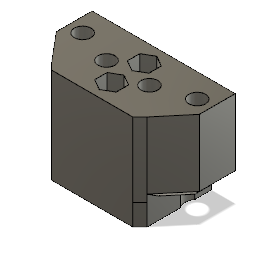
Hanger__Ceiling__Interchange (Autodesk Fusion 360 design; units mm, degrees)
Autodesk Fusion 360 part; units mm, degrees
sketch "Sketch1" plane through (0, 0, 0) normal (0, 1, 0) x (1, 0, 0)
  line L0 (0, 0) -> (60, 0)
  line L1 (60, 0) -> (60, -40)
  line L2 (60, -40) -> (0, -40)
  line L3 (0, -40) -> (0, 0)
  dimension "d1" = 60
  dimension "d2" = 40
  constraint horizontal L0
  constraint vertical L1
  constraint horizontal L2
  constraint vertical L3
  constraint coincident L0.start L3.end
  measures "d1" distance of L0.start L0.end
  measures "d2" distance of L0.start L2.end
extrude "Extrude1" add sketch "Sketch1" along normal blind 25
sketch "Sketch2" plane through (0, 25, 0) normal (0, 1, 0) x (-1, 0, 0)
  line L0 (0, 40) -> (-60, 40)
  line L1 (-60, 40) -> (-60, 0)
  line L2 (-60, 0) -> (0, 0)
  line L3 (0, 0) -> (0, 40)
  line L4 (-30, 0) -> (-30, 20)
  line L5 (-30, 20) -> (-39, 20)
  line L6 (-30, 20) -> (-21, 20)
  line L7 (-21, 20) -> (-6, 20)
  line L8 (-39, 20) -> (-54, 20)
  circle A0 centre (-21, 20) radius 3.5
  circle A1 centre (-39, 20) radius 3.5
  circle A2 centre (-54, 20) radius 3.5
  circle A3 centre (-6, 20) radius 3.5
  dimension "d5" = 20
  dimension "d6" = 9
  dimension "d7" = 9
  dimension "d8" = 15
  dimension "d9" = 15
  dimension "d10" = 7
  dimension "d11" = 7
  dimension "d12" = 7
  dimension "d13" = 7
  constraint midpoint L2 L4.start
  constraint perpendicular L0 L4
  constraint perpendicular L4 L5
  constraint perpendicular L4 L6
  constraint parallel L6 L7
  constraint perpendicular L4 L8
  constraint coincident L6.end L7.start
  constraint coincident L5.end L8.start
  constraint coincident L8.end A2.centre
  constraint coincident L7.end A3.centre
  measures "d5" distance of L4.start L4.end
  measures "d6" distance of L4.end L5.end
  measures "d7" distance of L4.end L6.end
  measures "d8" distance of L6.end L7.end
  measures "d9" distance of L5.end L8.end
  measures "d10" diameter of A0
  measures "d11" diameter of A1
  measures "d12" diameter of A2
  measures "d13" diameter of A3
extrude "Extrude2" cut sketch "Sketch2" against normal blind 25 contours L5 L8 A1 | L5 L8 A1 | L6 L7 A0 | L6 L7 A0 | A2 | A3
sketch "Sketch3" plane through (0, 0, 0) normal (0, -1, 0) x (1, 0, 0)
  circle A0 centre (21, 20) radius 3.5
  circle A1 centre (39, 20) radius 3.5
  circle A2 centre (6, 20) radius 3.5
  circle A3 centre (54, 20) radius 3.5
  line L0 (60, 40) -> (0, 40)
  line L1 (0, 40) -> (0, 0)
  line L2 (0, 0) -> (60, 0)
  line L3 (60, 0) -> (60, 40)
  circle A4 centre (6, 20) radius 6.5
  circle A5 centre (21, 20) radius 6.5
  circle A6 centre (39, 20) radius 6.5
  circle A7 centre (54, 20) radius 6.5
  dimension "d16" = 13
  dimension "d17" = 13
  dimension "d18" = 13
  dimension "d19" = 13
  constraint concentric A2 A4
  constraint concentric A0 A5
  constraint concentric A1 A6
  constraint concentric A3 A7
  measures "d16" diameter of A4
  measures "d17" diameter of A5
  measures "d18" diameter of A6
  measures "d19" diameter of A7
extrude "Extrude3" cut sketch "Sketch3" against normal blind 2 contours L3 A7 | L1 A4 | A5 | A6 picked at (59.1667, 20) picked at (0.8333, 20)
extrude "Extrude4" cut 4 faces at (0.8333, 2, 20) (26.4628, 2, 19.5032) (44.4758, 2, 19.6771) (59.1667, 2, 20) along direction (0, 1, 0) blind 13
sketch "Sketch4" plane through (0, 25, 0) normal (0, 1, 0) x (-1, 0, 0)
  circle A0 centre (-21, 20) radius 3.5
  circle A1 centre (-39, 20) radius 3.5
  circle A2 centre (-6, 20) radius 3.5
  circle A3 centre (-54, 20) radius 3.5
  line L0 (0, 40) -> (-60, 40)
  line L1 (-60, 40) -> (-60, 0)
  line L2 (-60, 0) -> (0, 0)
  line L3 (0, 0) -> (0, 40)
  line L4 (-30, 40) -> (-30, 0)
  line L5 (-30, 20) -> (-30, 26.85)
  line L6 (-30, 26.85) -> (-30, 13.15)
  circle A4 centre (-30, 13.15) radius 2
  circle A5 centre (-30, 26.85) radius 2
  dimension "d24" = 6.85
  dimension "d25" = 13.7
  dimension "d26" = 4
  dimension "d27" = 4
  constraint midpoint L0 L4.start
  constraint midpoint L2 L4.end
  constraint midpoint L4 L5.start
  constraint parallel L4 L5
  constraint parallel L4 L6
  constraint coincident L6.end A4.centre
  constraint coincident L5.end L6.start
  measures "d24" distance of L5.start L5.end
  measures "d25" distance of L5.end L6.end
  measures "d26" diameter of A4
  measures "d27" diameter of A5
sketch "Sketch5" plane through (0, 25, 0) normal (0, 1, 0) x (-1, 0, 0)
  circle A0 centre (-21, 20) radius 3.5
  circle A1 centre (-39, 20) radius 3.5
  circle A2 centre (-6, 20) radius 3.5
  circle A3 centre (-54, 20) radius 3.5
  line L0 (0, 40) -> (-60, 40)
  line L1 (-60, 40) -> (-60, 0)
  line L2 (-60, 0) -> (0, 0)
  line L3 (0, 0) -> (0, 40)
  line L4 (-34.5, 24.2519) -> (-30, 21.6538)
  line L5 (-30, 21.6538) -> (-25.5, 24.2519)
  line L6 (-25.5, 24.2519) -> (-25.5, 29.4481)
  line L7 (-25.5, 29.4481) -> (-30, 32.0462)
  line L8 (-30, 32.0462) -> (-34.5, 29.4481)
  line L9 (-34.5, 29.4481) -> (-34.5, 24.2519)
  line L10 (-34.5, 10.5519) -> (-30, 7.9538)
  line L11 (-30, 7.9538) -> (-25.5, 10.5519)
  line L12 (-25.5, 10.5519) -> (-25.5, 15.7481)
  line L13 (-25.5, 15.7481) -> (-30, 18.3462)
  line L14 (-30, 18.3462) -> (-34.5, 15.7481)
  line L15 (-34.5, 15.7481) -> (-34.5, 10.5519)
  point P0 (-30, 26.85)
  point P1 (-30, 13.15)
  dimension "d30" = 4.5
  dimension "d31" = 4.5
  measures "d30" distance of P0 L9
  measures "d31" distance of P1 L15
sketch "Sketch6" plane through (0, 0, 0) normal (0, -1, 0) x (1, 0, 0)
  arc A0 (60, 22.5) -> (60, 17.5) centre (54, 20) ccw
  line L0 (60, 22.5) -> (60, 40)
  line L1 (60, 40) -> (0, 40)
  line L2 (0, 40) -> (0, 22.5)
  arc A1 (0, 17.5) -> (0, 22.5) centre (6, 20) ccw
  line L3 (0, 17.5) -> (0, 0)
  line L4 (0, 0) -> (60, 0)
  line L5 (60, 0) -> (60, 17.5)
  circle A2 centre (21, 20) radius 6.5
  circle A3 centre (39, 20) radius 6.5
  circle A4 centre (6, 20) radius 5
  circle A5 centre (21, 20) radius 5
  circle A6 centre (54, 20) radius 5
  circle A7 centre (39, 20) radius 5
  circle A8 centre (6, 20) radius 6.5
  circle A9 centre (54, 20) radius 6.5
  circle A10 centre (39, 20) radius 6.5
  circle A11 centre (21, 20) radius 6.5
  dimension "d32" = 10
  dimension "d33" = 10
  dimension "d34" = 10
  dimension "d35" = 10
  constraint concentric A1 A4
  constraint concentric A2 A5
  constraint concentric A0 A6
  constraint concentric A3 A7
  constraint concentric A4 A8
  constraint concentric A6 A9
  constraint concentric A7 A10
  constraint concentric A5 A11
  measures "d32" diameter of A4
  measures "d33" diameter of A5
  measures "d34" diameter of A6
  measures "d35" diameter of A7
extrude "Extrude6" add sketch "Sketch6" against normal blind 15 contours A0 A9 | A1 A8 | A2 A11 | A3 A10
sketch "Sketch7" plane through (0, 25, 0) normal (0, 1, 0) x (-1, 0, 0)
  circle A0 centre (-21, 20) radius 3.5
  circle A1 centre (-39, 20) radius 3.5
  circle A2 centre (-6, 20) radius 3.5
  circle A3 centre (-54, 20) radius 3.5
  line L0 (0, 40) -> (-60, 40)
  line L1 (-60, 40) -> (-60, 0)
  line L2 (-60, 0) -> (0, 0)
  line L3 (0, 0) -> (0, 40)
  line L4 (-60, 40) -> (0, 40)
  line L5 (0, 40) -> (0, 0)
  line L6 (0, 0) -> (-60, 0)
  line L7 (-60, 0) -> (-60, 40)
  line L8 (-63.5098, 43.7878) -> (2.9374, 43.7878)
  line L9 (2.9374, 43.7878) -> (2.9374, -3.4155)
  line L10 (2.9374, -3.4155) -> (-63.5098, -3.4155)
  line L11 (-63.5098, -3.4155) -> (-63.5098, 43.7878)
  constraint horizontal L4
  constraint vertical L5
  constraint horizontal L6
  constraint vertical L7
  constraint coincident L2.end L3.start
  constraint coincident L0.end L1.start
  constraint horizontal L8
  constraint vertical L9
  constraint horizontal L10
  constraint vertical L11
extrude "Extrude8" cut sketch "Sketch7" against normal blind 41 contours L8 L9 L10 L11
sketch "Sketch8" plane through (0, 0, 0) normal (-1, 0, 0) x (0, 0, 1)
  line L0 (0, 0) -> (40, 0)
  line L1 (40, 0) -> (40, 25)
  line L2 (40, 25) -> (0, 25)
  line L3 (0, 25) -> (0, 0)
  line L4 (40, 0) -> (37, 0)
  line L5 (40, 0) -> (40, 3)
  line L6 (40, 3) -> (37, 0)
  dimension "d42" = 3
  dimension "d43" = 3
  constraint coincident L0.end L1.start
  constraint perpendicular L1 L4
  constraint perpendicular L0 L5
  measures "d42" distance of L0.end L4.end
  measures "d43" distance of L0.end L5.end
extrude "Extrude9" cut sketch "Sketch8" against normal blind 10 contours L0 L1 L4 L5 L6
extrude "Extrude10" cut 1 faces at (10, 1, 39) along direction (-1, 0, 0) blind -40 and the other way blind 50
sketch "Sketch9" plane through (0, 25, 0) normal (0, 1, 0) x (-1, 0, 0)
  circle A0 centre (-21, 20) radius 3.5
  circle A1 centre (-39, 20) radius 3.5
  circle A2 centre (-6, 20) radius 3.5
  circle A3 centre (-54, 20) radius 3.5
  line L0 (0, 40) -> (-60, 40)
  line L1 (-60, 40) -> (-60, 0)
  line L2 (-60, 0) -> (0, 0)
  line L3 (0, 0) -> (0, 40)
  line L4 (-30, 40) -> (-30, 31.85)
  circle A4 centre (-30, 31.85) radius 2
  line L5 (-30, 31.85) -> (-30, 18.15)
  circle A5 centre (-30, 18.15) radius 2
  dimension "d50" = 8.15
  dimension "d51" = 4
  dimension "d52" = 13.7
  dimension "d53" = 4
  constraint midpoint L0 L4.start
  constraint perpendicular L0 L4
  constraint coincident L4.end A4.centre
  constraint parallel L4 L5
  constraint coincident L5.end A5.centre
  measures "d50" distance of L4.start L4.end
  measures "d51" diameter of A4
  measures "d52" distance of L4.end L5.end
  measures "d53" diameter of A5
extrude "Extrude11" cut sketch "Sketch9" against normal blind 25 contours L4 A4 L5 | L4 A4 L5 | A5
sketch "Sketch10" plane through (0, 25, 0) normal (0, 1, 0) x (-1, 0, 0)
  circle A0 centre (-30, 31.85) radius 2
  circle A1 centre (-30, 18.15) radius 2
  circle A2 centre (-21, 20) radius 3.5
  circle A3 centre (-39, 20) radius 3.5
  circle A4 centre (-6, 20) radius 3.5
  circle A5 centre (-54, 20) radius 3.5
  line L0 (0, 40) -> (-60, 40)
  line L1 (-60, 40) -> (-60, 0)
  line L2 (-60, 0) -> (0, 0)
  line L3 (0, 0) -> (0, 40)
  line L4 (-34.5, 29.2519) -> (-30, 26.6538)
  line L5 (-30, 26.6538) -> (-25.5, 29.2519)
  line L6 (-25.5, 29.2519) -> (-25.5, 34.4481)
  line L7 (-25.5, 34.4481) -> (-30, 37.0462)
  line L8 (-30, 37.0462) -> (-34.5, 34.4481)
  line L9 (-34.5, 34.4481) -> (-34.5, 29.2519)
  line L10 (-34.5, 15.5519) -> (-30, 12.9538)
  line L11 (-30, 12.9538) -> (-25.5, 15.5519)
  line L12 (-25.5, 15.5519) -> (-25.5, 20.7481)
  line L13 (-25.5, 20.7481) -> (-30, 23.3462)
  line L14 (-30, 23.3462) -> (-34.5, 20.7481)
  line L15 (-34.5, 20.7481) -> (-34.5, 15.5519)
  point P0 (-30, 31.85)
  point P1 (-30, 18.15)
  dimension "d56" = 4.5
  dimension "d57" = 4.5
  constraint coincident P0 A0.centre
  constraint coincident P1 A1.centre
  measures "d56" distance of P0 L9
  measures "d57" distance of P1 L15
extrude "Extrude12" cut sketch "Sketch10" against normal blind 15 contours L4 L5 L6 L7 L8 L9 | L10 L11 L12 L13 L14 L15
sketch "Sketch11" plane through (0, 0, 0) normal (0, -1, 0) x (1, 0, 0)
sketch "Sketch12" plane through (0, 0, 40) normal (0, 0, 1) x (1, 0, 0)
sketch "Sketch13" plane through (0, 0, 0) normal (0, -1, 0) x (1, 0, 0)
sketch "Sketch14" plane through (0, 0, 40) normal (0, 0, 1) x (1, 0, 0)
ref_plane "WorkPlane1" through (11.5, 0, 38.5) normal (-0.579228, -0.573576, 0.579228) x (-0.707107, 0, -0.707107)
sketch "Sketch15" plane through (11.5, 0, 38.5) normal (-0.579228, -0.573576, 0.579228) x (-0.707107, 0, -0.707107)
  line L0 (2.1213, 0, 0) -> (0, -3.6742, 0.017)
  line L1 (0, -3.6742, 0.017) -> (-2.1213, 0, 0)
  line L2 (-2.1213, 0) -> (2.1213, 0)
  point P0 (2.1213, 0)
  point P1 (0, -3.6742)
  point P2 (-2.1213, 0)
  constraint coincident P0 L2.end
  constraint coincident P2 L2.start
extrude "Extrude13" cut sketch "Sketch15" along normal blind 5 contours L0 L1 L2 in plane through (11.5, 0, 38.5) normal (-0.57735, -0.57735, 0.57735)
ref_plane "WorkPlane2" through (48.5, 1.5, 40) normal (0.579228, -0.579228, 0.573576) x (0.707107, 0.707107, 0)
sketch "Sketch16" plane through (48.5, 1.5, 40) normal (0.579228, -0.579228, 0.573576) x (0.707107, 0.707107, 0)
  line L0 (-2.1213, 0) -> (2.1213, 0)
  line L1 (2.1213, 0, 0) -> (0, -3.6742, 0.017)
  line L2 (0, -3.6742, 0.017) -> (-2.1213, 0, 0)
  point P0 (-2.1213, 0)
  point P1 (2.1213, 0)
  point P2 (0, -3.6742)
  constraint coincident P0 L0.start
  constraint coincident P1 L0.end
extrude "Extrude14" cut sketch "Sketch16" along normal blind 5 contours L0 L1 L2 in plane through (48.5, 1.5, 40) normal (0.57735, -0.57735, 0.57735)
chamfer "Chamfer1" distance 3 distance2 3 2 edges at (0, 14, 40) (60, 14, 40) measured on face at (0, 16.6667, 25.6667) measured on face at (23.3333, 17.6667, 40)
chamfer "Chamfer2" distance 3 angle 45 1 edges at (60, 0, 18.5)
chamfer "Chamfer3" distance 3 angle 45 1 edges at (0, 0, 18.5)
extrude "Extrude15" add 1 faces at (30, 25, 4.3179) along direction (0, 1, 0) blind 15
extrude "Extrude16" add 2 faces at (28.1667, 10, 28.6746) (28.1667, 10, 14.9746) along direction (0, 1, 0) blind 15
extrude "Extrude17" cut 4 faces at (10.4684, 15, 19.5777) (25.1536, 15, 19.349) (34.8464, 15, 19.349) (58.4684, 15, 19.5777) along direction (0, 1, 0) blind 15
extrude "Extrude18" cut 1 faces at (39, 26.6667, 0) along direction (0, 0, 1) blind 5
sketch "Sketch17" plane through (0, 0, 0) normal (0, -1, 0) x (1, 0, 0)
  line L0 (3, 5) -> (57, 5)
  line L1 (57, 5) -> (57, 16)
  arc A0 (57, 24) -> (57, 16) centre (54, 20) ccw
  line L2 (57, 24) -> (57, 37)
  line L3 (57, 37) -> (50, 37)
  line L4 (50, 37) -> (47, 40)
  line L5 (47, 40) -> (13, 40)
  line L6 (13, 40) -> (10, 37)
  line L7 (10, 37) -> (3, 37)
  line L8 (3, 37) -> (3, 24)
  arc A1 (3, 16) -> (3, 24) centre (6, 20) ccw
  line L9 (3, 16) -> (3, 5)
  circle A2 centre (30, 31.85) radius 2
  circle A3 centre (30, 18.15) radius 2
  circle A4 centre (21, 20) radius 5
  circle A5 centre (39, 20) radius 5
  line L10 (50, 37) -> (50, 54.6936)
  line L11 (50, 37) -> (50, 40)
  line L12 (50, 40) -> (62.2647, 25.3835)
  line L13 (62.2647, 25.3835) -> (62.2647, 41)
  line L14 (62.2647, 41) -> (50, 41)
  line L15 (10, 37) -> (10, 40)
  line L16 (10, 40) -> (-2.3313, 25.3041)
  line L17 (-2.3313, 25.3041) -> (-2.3313, 43)
  line L18 (-2.3313, 43) -> (10, 43)
  line L19 (10, 43) -> (10, 40)
  dimension "d81" = 40
  dimension "d82" = 40
  constraint coincident L3.end L4.start
  constraint perpendicular L3 L10
  constraint coincident L10 L11.end
  constraint parallel L11 L13
  constraint coincident L10 L14.end
  constraint perpendicular L10 L14
  constraint coincident L6.end L7.start
  constraint perpendicular L7 L15
  constraint perpendicular L7 L17
  constraint perpendicular L15 L18
  constraint perpendicular L18 L19
  measures "d81" angle of L11 L12
  measures "d82" angle of L15 L16
extrude "Extrude19" cut sketch "Sketch17" against normal blind 50 contours L7 L8 L16 L17 L18 L19 | L7 L8 L16 | L2 L3 L12 | L2 L3 L10 L12 L13 L14
sketch "Sketch18" plane through (60, 0, 0) normal (1, 0, 0) x (0, 0, -1)
  line L0 (-28.0825, 40) -> (-28.0825, 3)
  line L1 (-28.0825, 3) -> (-5, 3)
  line L2 (-5, 3) -> (-5, 40)
  line L3 (-5, 40) -> (-28.0825, 40)
  line L4 (-5, 0) -> (-40, 0)
  line L5 (-40, 0) -> (-40, 9)
  line L6 (-40, 9) -> (-5, 9)
  line L7 (-5, 9) -> (-5, 0)
  dimension "d85" = 9
  constraint horizontal L4
  constraint vertical L5
  constraint horizontal L6
  constraint vertical L7
  measures "d85" distance of L4.start L6.end
extrude "Extrude20" cut sketch "Sketch18" against normal blind 5 contours L0 L1 L2 L6 L7 | L0 L1 L4 L5 L6 L7
sketch "Sketch19" plane through (0, 0, 0) normal (-1, 0, 0) x (0, 0, 1)
  line L0 (28.0825, 3) -> (28.0825, 40)
  line L1 (28.0825, 40) -> (5, 40)
  line L2 (5, 40) -> (5, 3)
  line L3 (5, 3) -> (28.0825, 3)
  line L4 (5, 0) -> (40, 0)
  line L5 (40, 0) -> (40, 9)
  line L6 (40, 9) -> (5, 9)
  line L7 (5, 9) -> (5, 0)
  dimension "d88" = 35
  dimension "d89" = 9
  constraint horizontal L4
  constraint vertical L5
  constraint horizontal L6
  constraint vertical L7
  measures "d88" distance of L4.start L4.end
  measures "d89" distance of L4.start L6.end
extrude "Extrude21" cut sketch "Sketch19" against normal blind 5 contours L0 L2 L3 L6 L7 | L0 L3 L4 L5 L6 L7
sketch "Sketch20" plane through (0, 0, 0) normal (0, -1, 0) x (1, 0, 0)
  line L0 (5, 15.101) -> (5, 5)
  line L1 (5, 5) -> (55, 5)
  line L2 (55, 5) -> (55, 15.101)
  arc A0 (55, 24.899) -> (55, 15.101) centre (54, 20) ccw
  line L3 (55, 24.899) -> (55, 34.0412)
  line L4 (55, 34.0412) -> (52.5173, 37)
  line L5 (52.5173, 37) -> (50, 37)
  line L6 (50, 37) -> (47, 40)
  line L7 (47, 40) -> (13, 40)
  line L8 (13, 40) -> (10, 37)
  line L9 (10, 37) -> (7.4827, 37)
  line L10 (7.4827, 37) -> (5, 34.0412)
  line L11 (5, 34.0412) -> (5, 24.899)
  arc A1 (5, 15.101) -> (5, 24.899) centre (6, 20) ccw
  circle A2 centre (30, 31.85) radius 2
  circle A3 centre (30, 18.15) radius 2
  circle A4 centre (21, 20) radius 5
  circle A5 centre (39, 20) radius 5
  line L12 (50, 37) -> (50, 5)
  line L13 (10, 37) -> (10, 5)
  line L14 (10, 5) -> (2, 5)
  line L15 (2, 5) -> (2, 40)
  line L16 (2, 40) -> (10, 40)
  line L17 (10, 40) -> (10, 5)
  line L18 (50, 5) -> (57, 5)
  line L19 (57, 5) -> (57, 40)
  line L20 (57, 40) -> (50, 40)
  line L21 (50, 40) -> (50, 5)
  constraint coincident L5.end L6.start
  constraint coincident L1 L12.end
  constraint perpendicular L1 L12
  constraint coincident L8.end L9.start
  constraint coincident L1 L13.end
  constraint perpendicular L1 L13
  constraint horizontal L14
  constraint vertical L15
  constraint horizontal L16
  constraint vertical L17
  constraint horizontal L18
  constraint vertical L19
  constraint horizontal L20
  constraint vertical L21
extrude "Extrude22" cut sketch "Sketch20" against normal blind 9 contours L0 L1 A1 L13 L14 L17 | L0 L9 L10 L11 A1 L13 L14 L15 L16 L17 | L9 L10 L11 A1 L13 L17 | L1 L2 A0 L12 L18 L21 | L2 A0 L3 L4 L5 L12 L18 L19 L20 L21 | A0 L3 L4 L5 L12 L21
sketch "Sketch21" plane through (0, 0, 40) normal (0, 0, 1) x (1, 0, 0)
  line L0 (10, 40) -> (10, 9)
  line L1 (10, 9) -> (10, 3)
  line L2 (10, 3) -> (13, 0)
  line L3 (13, 0) -> (47, 0)
  line L4 (47, 0) -> (50, 3)
  line L5 (50, 3) -> (50, 9)
  line L6 (50, 9) -> (50, 40)
  line L7 (50, 40) -> (10, 40)
  line L8 (10, 0) -> (14, 0)
  line L9 (14, 0) -> (14, 3)
  line L10 (14, 3) -> (10, 3)
  line L11 (10, 3) -> (10, 0)
  line L12 (50, 0) -> (47, 0)
  line L13 (47, 0) -> (47, 3.1875)
  line L14 (47, 3.1875) -> (50, 3.1875)
  line L15 (50, 3.1875) -> (50, 0)
  constraint horizontal L8
  constraint vertical L9
  constraint horizontal L10
  constraint vertical L11
  constraint horizontal L12
  constraint vertical L13
  constraint horizontal L14
  constraint vertical L15
extrude "Extrude23" add sketch "Sketch21" against normal blind 3 contours L2 L8 L11 | L4 L12 L15
chamfer "Chamfer5" distance 3 angle 45 2 edges at (10, 4.5, 40) (50, 4.5, 40)
sketch "Sketch22" plane through (0, 0, 0) normal (0, -1, 0) x (1, 0, 0)
  circle A0 centre (39, 20) radius 5
  circle A1 centre (21, 20) radius 5
  circle A2 centre (30, 18.15) radius 2
  circle A3 centre (30, 31.85) radius 2
  line L0 (50, 37) -> (47, 40)
  line L1 (47, 40) -> (13, 40)
  line L2 (13, 40) -> (10, 37)
  line L3 (10, 37) -> (10, 23)
  arc A4 (10, 17) -> (10, 23) centre (6, 20) ccw
  line L4 (10, 17) -> (10, 5)
  line L5 (10, 5) -> (50, 5)
  line L6 (50, 5) -> (50, 17)
  arc A5 (50, 23) -> (50, 17) centre (54, 20) ccw
  line L7 (50, 23) -> (50, 37)
  line L8 (10, 37) -> (0, 28)
  line L9 (50, 37) -> (60, 28)
  line L10 (0, 28) -> (60, 28)
  line L11 (60, 28) -> (60, 40)
  line L12 (60, 40) -> (0, 40)
  line L13 (0, 40) -> (0, 28)
  line L14 (10, 37) -> (13, 37)
  line L15 (13, 37) -> (13, 40)
  line L16 (13, 40) -> (10, 40)
  line L17 (10, 40) -> (10, 37)
  line L18 (50, 37) -> (47, 37)
  line L19 (47, 37) -> (47, 40)
  line L20 (47, 40) -> (50, 40)
  line L21 (50, 40) -> (50, 37)
  constraint coincident L2.end L3.start
  constraint coincident L0.start L7.end
  constraint horizontal L10
  constraint vertical L11
  constraint horizontal L12
  constraint vertical L13
  constraint horizontal L14
  constraint vertical L15
  constraint horizontal L16
  constraint vertical L17
  constraint coincident L1.end L2.start
  constraint horizontal L18
  constraint vertical L19
  constraint horizontal L20
  constraint vertical L21
  constraint coincident L0.end L1.start
extrude "Extrude24" cut sketch "Sketch22" against normal blind 100 contours L9 L11 L12 L21 | L0 L12 L20 L21 | L2 L12 L16 L17 | L8 L12 L13 L17
sketch "Sketch23" plane through (0, 0, 0) normal (0, -1, 0) x (1, 0, 0)
  circle A0 centre (39, 20) radius 5
  circle A1 centre (21, 20) radius 5
  circle A2 centre (30, 18.15) radius 2
  circle A3 centre (30, 31.85) radius 2
  line L0 (50, 37) -> (47, 40)
  line L1 (47, 40) -> (13, 40)
  line L2 (13, 40) -> (10, 37)
  line L3 (10, 37) -> (10, 23)
  arc A4 (10, 17) -> (10, 23) centre (6, 20) ccw
  line L4 (10, 17) -> (10, 5)
  line L5 (10, 5) -> (50, 5)
  line L6 (50, 5) -> (50, 17)
  arc A5 (50, 23) -> (50, 17) centre (54, 20) ccw
  line L7 (50, 23) -> (50, 37)
  line L8 (50, 37) -> (62.7874, 21.7606)
  line L9 (50, 37) -> (69.8936, 37) construction
  line L10 (10, 37) -> (-2.0257, 22.6684)
  line L11 (10, 37) -> (28.7086, 37) construction
  line L12 (-2.0257, 22.6684) -> (62.7874, 22.6684)
  line L13 (62.7874, 22.6684) -> (62.7874, 45.0578)
  line L14 (62.7874, 45.0578) -> (-2.0257, 45.0578)
  line L15 (-2.0257, 45.0578) -> (-2.0257, 22.6684)
  dimension "d102" = 50
  dimension "d103" = 130
  constraint horizontal L9
  constraint coincident L0.start L7.end
  constraint horizontal L11
  constraint coincident L2.end L3.start
  constraint horizontal L12
  constraint vertical L13
  constraint horizontal L14
  constraint vertical L15
  measures "d102" angle of L8 L9
  measures "d103" angle of L10 L11
extrude "Extrude25" cut sketch "Sketch23" against normal blind 50 contours L0 L1 L2 L8 L10 L12 L13 L14 L15
chamfer "Chamfer9" distance 3 angle 45 4 edges at (55, 9, 31.0412) (60, 9, 15.0412) (5, 9, 31.0412) (0, 9, 15.0412)
extrude "Extrude32" cut 1 faces at (36.6667, 29.6667, 5) along direction (0, 0, 1) blind 5
sketch "Sketch29" plane through (0, 40, 0) normal (0, 1, 0) x (-1, 0, 0)
  circle A0 centre (-54, 20) radius 3.5
  circle A1 centre (-6, 20) radius 3.5
  circle A2 centre (-39, 20) radius 3.5
  circle A3 centre (-21, 20) radius 3.5
  line L0 (-30, 12.9538) -> (-34.5, 15.5519)
  line L1 (-34.5, 15.5519) -> (-34.5, 20.7481)
  line L2 (-34.5, 20.7481) -> (-30, 23.3462)
  line L3 (-30, 23.3462) -> (-25.5, 20.7481)
  line L4 (-25.5, 20.7481) -> (-25.5, 15.5519)
  line L5 (-25.5, 15.5519) -> (-30, 12.9538)
  line L6 (-30, 26.6538) -> (-34.5, 29.2519)
  line L7 (-34.5, 29.2519) -> (-34.5, 34.4481)
  line L8 (-34.5, 34.4481) -> (-30, 37.0462)
  line L9 (-30, 37.0462) -> (-25.5, 34.4481)
  line L10 (-25.5, 34.4481) -> (-25.5, 29.2519)
  line L11 (-25.5, 29.2519) -> (-30, 26.6538)
  line L12 (-60, 10) -> (0, 10)
  line L13 (0, 10) -> (0, 25.0825)
  line L14 (0, 25.0825) -> (-10, 37)
  line L15 (-10, 37) -> (-13, 40)
  line L16 (-13, 40) -> (-47, 40)
  line L17 (-47, 40) -> (-50, 37)
  line L18 (-50, 37) -> (-60, 25.0825)
  line L19 (-60, 25.0825) -> (-60, 10)
  circle A4 centre (-39, 20) radius 3.5
  circle A5 centre (-21, 20) radius 3.5
  constraint concentric A2 A4
  constraint concentric A3 A5
extrude "Extrude33" add sketch "Sketch29" against normal blind 40 contours A2 A4 | A3 A5
extrude "Extrude34" add 2 faces at (34.8464, 30, 19.349) (25.1536, 30, 19.349) along direction (0, -1, 0) blind 30
sketch "Sketch30" plane through (0, 0, 0) normal (0, -1, 0) x (1, 0, 0)
  line L0 (10, 10) -> (50, 10)
  line L1 (50, 10) -> (50, 17)
  arc A0 (50, 23) -> (50, 17) centre (54, 20) ccw
  line L2 (50, 23) -> (50, 37)
  line L3 (50, 37) -> (47, 40)
  line L4 (47, 40) -> (13, 40)
  line L5 (13, 40) -> (10, 37)
  line L6 (10, 37) -> (10, 23)
  arc A1 (10, 17) -> (10, 23) centre (6, 20) ccw
  line L7 (10, 17) -> (10, 10)
  arc A2 (34.0971, 20.9807) -> (34.5, 17.8206) centre (39, 20) ccw
  line L8 (34.0971, 20.9807) -> (34.5, 20.7481)
  line L9 (34.5, 20.7481) -> (34.5, 17.8206)
  arc A3 (25.5, 17.8206) -> (25.9029, 20.9807) centre (21, 20) ccw
  line L10 (25.5, 17.8206) -> (25.5, 20.7481)
  line L11 (25.5, 20.7481) -> (25.9029, 20.9807)
  circle A4 centre (30, 18.15) radius 2
  circle A5 centre (30, 31.85) radius 2
  line L12 (33, 16) -> (36, 16)
  line L13 (36, 16) -> (36, 22)
  line L14 (36, 22) -> (33, 22)
  line L15 (33, 22) -> (33, 16)
  line L16 (27, 22) -> (24, 22)
  line L17 (24, 22) -> (24, 16)
  line L18 (24, 16) -> (27, 16)
  line L19 (27, 16) -> (27, 22)
  constraint horizontal L12
  constraint vertical L13
  constraint horizontal L14
  constraint vertical L15
  constraint horizontal L16
  constraint vertical L17
  constraint horizontal L18
  constraint vertical L19
extrude "Extrude35" add sketch "Sketch30" against normal blind 25 contours A2 L8 L9 | A3 L10 L11
sketch "Sketch31" plane through (0, 40, 0) normal (0, 1, 0) x (-1, 0, 0)
  circle A0 centre (-54, 20) radius 3.5
  circle A1 centre (-6, 20) radius 3.5
  line L0 (-30, 12.9538) -> (-34.5, 15.5519)
  line L1 (-34.5, 15.5519) -> (-34.5, 20.7481)
  line L2 (-34.5, 20.7481) -> (-30, 23.3462)
  line L3 (-30, 23.3462) -> (-25.5, 20.7481)
  line L4 (-25.5, 20.7481) -> (-25.5, 15.5519)
  line L5 (-25.5, 15.5519) -> (-30, 12.9538)
  line L6 (-30, 26.6538) -> (-34.5, 29.2519)
  line L7 (-34.5, 29.2519) -> (-34.5, 34.4481)
  line L8 (-34.5, 34.4481) -> (-30, 37.0462)
  line L9 (-30, 37.0462) -> (-25.5, 34.4481)
  line L10 (-25.5, 34.4481) -> (-25.5, 29.2519)
  line L11 (-25.5, 29.2519) -> (-30, 26.6538)
  line L12 (-60, 10) -> (0, 10)
  line L13 (0, 10) -> (0, 25.0825)
  line L14 (0, 25.0825) -> (-10, 37)
  line L15 (-10, 37) -> (-13, 40)
  line L16 (-13, 40) -> (-47, 40)
  line L17 (-47, 40) -> (-50, 37)
  line L18 (-50, 37) -> (-60, 25.0825)
  line L19 (-60, 25.0825) -> (-60, 10)
  line L20 (-30, 23.3462) -> (-30, 26.6538)
  line L21 (-30, 25) -> (-39, 25)
  line L22 (-30, 25) -> (-21, 25)
  circle A2 centre (-39, 25) radius 3.5
  circle A3 centre (-21, 25) radius 3.5
  dimension "d139" = 9
  dimension "d140" = 9
  dimension "d141" = 7
  dimension "d142" = 7
  constraint coincident L2.end L3.start
  constraint coincident L6.start L11.end
  constraint midpoint L20 L21.start
  constraint perpendicular L20 L21
  constraint perpendicular L20 L22
  constraint coincident L21.end A2.centre
  constraint coincident L22.end A3.centre
  measures "d139" distance of L21.start L21.end
  measures "d140" distance of L21.start L22.end
  measures "d141" diameter of A2
  measures "d142" diameter of A3
extrude "Extrude36" cut sketch "Sketch31" against normal blind 30 contours A2 | A3
extrude "Extrude37" cut 2 faces at (38.3114, 10, 25.7421) (22.0511, 10, 25.5062) along direction (0, -1, 0) blind 30
sketch "Sketch32" plane through (0, 0, 0) normal (0, -1, 0) x (1, 0, 0)
  circle A0 centre (39, 25) radius 3.5
  circle A1 centre (21, 25) radius 3.5
  line L0 (10, 10) -> (50, 10)
  line L1 (50, 10) -> (50, 17)
  arc A2 (50, 23) -> (50, 17) centre (54, 20) ccw
  line L2 (50, 23) -> (50, 37)
  line L3 (50, 37) -> (47, 40)
  line L4 (47, 40) -> (13, 40)
  line L5 (13, 40) -> (10, 37)
  line L6 (10, 37) -> (10, 23)
  arc A3 (10, 17) -> (10, 23) centre (6, 20) ccw
  line L7 (10, 17) -> (10, 10)
  circle A4 centre (30, 18.15) radius 2
  circle A5 centre (30, 31.85) radius 2
  circle A6 centre (39, 25) radius 5
  circle A7 centre (21, 25) radius 5
  dimension "d147" = 10
  constraint concentric A0 A6
  constraint concentric A1 A7
  measures "d147" diameter of A7
extrude "Extrude38" cut sketch "Sketch32" against normal blind 30 contours A6 | A7
